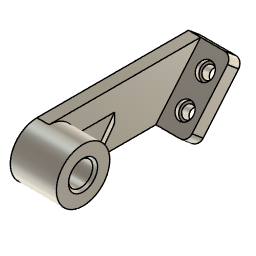
19 (Autodesk Fusion 360 design; units mm, degrees)
Autodesk Fusion 360 part; units mm, degrees
sketch "草图1" plane through (0, 0, 0) normal (1, 0, 0) x (0, 1, 0)
  circle A0 centre (0, 0) radius 5
  circle A1 centre (0, 0) radius 11
  line L0 (0, 11) -> (62.4602, 11)
  line L1 (62.4602, 11) -> (44, -11)
  line L2 (44, -11) -> (0, -11)
  line L3 (62.4602, 11) -> (67.0565, 7.1433)
  line L4 (67.0565, 7.1433) -> (48.5963, -14.8567)
  line L5 (48.5963, -14.8567) -> (44, -11)
  dimension "d1" = 22
  dimension "d2" = 10
  dimension "d3" = 44
  dimension "d4" = 130
  dimension "d5" = 6
  constraint coincident A0.centre A1.centre
  constraint coincident A1 L0.start
  constraint tangent A1 L0
  constraint horizontal L0
  constraint coincident A1 L2.end
  constraint tangent A1 L2
  constraint parallel L0 L2
  constraint perpendicular L1 L3
  constraint perpendicular L3 L4
  constraint parallel L3 L5
  measures "d1" diameter of A1
  measures "d2" diameter of A0
  measures "d3" distance of L1.end L2.end
  measures "d4" angle of L1 L2
  measures "d5" distance of L0.end L3.end
extrude "拉伸1" add sketch "草图1" along normal blind 19 contours A1 makes body 1
extrude "拉伸2" add sketch "草图1" along normal blind 5 contours A1 L0 L1 L2 bodies 1
extrude "拉伸3" add sketch "草图1" along normal blind 18 contours L1 L3 L4 L5 bodies 1
fillet "圆角1" radius 3 2 edges at (18, 64.7583, 9.0716) (18, 46.2981, -12.9284) on bodies 1
chamfer "倒角1" distance 1 angle 45 1 edges at (19, -4.6616, 1.8081) on bodies 1
sketch "草图2" plane through (0, 31.2367, -26.2107) normal (0, -0.766044, 0.642788) x (1, 0, 0)
  arc A0 (15, 19.8562) -> (18, 22.8562) centre (15, 22.8562) ccw
  line L0 (18, 22.8562) -> (18, 45.5751)
  arc A1 (18, 45.5751) -> (15, 48.5751) centre (15, 45.5751) ccw
  line L1 (15, 48.5751) -> (5, 48.5751)
  line L2 (5, 48.5751) -> (5, 19.8562)
  line L3 (5, 19.8562) -> (15, 19.8562)
  line L4 (18, 34.2156) -> (5, 34.2156) construction
  circle A2 centre (12, 40.7156) radius 3.5
  circle A3 centre (12, 40.7156) radius 2.5
  circle A4 centre (12, 27.7156) radius 3.5
  circle A5 centre (12, 27.7156) radius 2.5
  dimension "d15" = 7
  dimension "d16" = 5
  dimension "d17" = 6
  dimension "d18" = 13
  constraint midpoint L0 L4.start
  constraint midpoint L2 L4.end
  constraint concentric A2 A3
  constraint concentric A4 A5
  constraint equal A3 A5
  constraint equal A2 A4
  constraint symmetric L4 A2.centre A4.centre
  measures "d15" diameter of A2
  measures "d16" diameter of A3
  measures "d17" distance of L0 A2.centre
  measures "d18" distance of A2.centre A4.centre
extrude "拉伸4" cut sketch "草图2" against normal blind 2 contours A2 | A4 bodies 1
extrude "拉伸5" cut 2 faces at (13.1784, 57.6864, 5.3108) (12.6885, 49.3537, -4.6197) along direction (0, 0.766044, -0.642788) blind 50 on bodies 1 bodies 1
sketch "草图3" plane through (0, 0, 0) normal (0, 0, 1) x (1, 0, 0)
  line L0 (5, 27) -> (20.5885, 0)
  line L1 (20.5885, 0) -> (5, 0)
  line L2 (5, 0) -> (5, 27)
  dimension "d23" = 5
  dimension "d24" = 27
  dimension "d25" = 30
  constraint horizontal L1
  constraint perpendicular L1 L2
  constraint collinear origin L0.end L1.end
  measures "d23" distance of origin L1.end
  measures "d24" distance of L0.start L1.end
  measures "d25" angle of L0 L2
extrude "拉伸6" add sketch "草图3" along normal mid plane 4 separate body makes body 2
extrude "拉伸7" cut sketch "草图1" along normal blind 43 contours A0 bodies 2
combine "合并1" operation add target body 1 tool bodies 2
